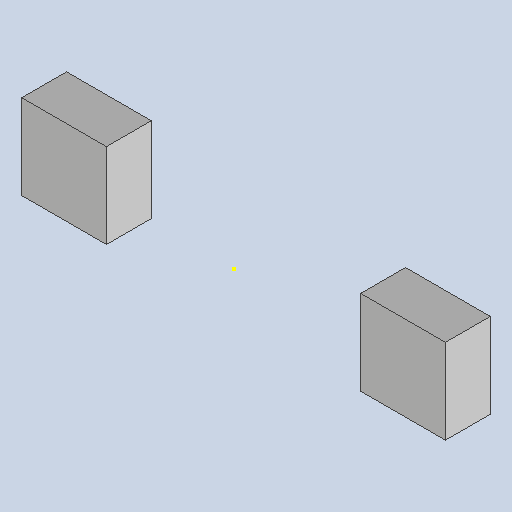
# Autodesk Inventor part: Dots2
Saved by Autodesk Inventor 2024.2 (Build 282272000, 272)
## iProperties
Created: 2024-01-22
Part Number: Dots2
Material: Generic
Document SubType Name: Modeling
Designer: Felix
Density: 1 g/cm^3
Appearance: Default
Author: Felix
Autodesk Inventor part; units mm, degrees
ref_plane "YZ Plane" through (0, 0, 0) normal (1, 0, 0) x (0, 1, 0)
ref_plane "XZ Plane" through (0, 0, 0) normal (0, 1, 0) x (-1, 0, 0)
ref_plane "XY Plane" through (0, 0, 0) normal (0, 0, 1) x (1, 0, 0)
sketch "Sketch1" plane through (0, 0, 0) normal (0, 1, 0) x (-1, 0, 0)
  point P0 (0, 0)
sketch "Sketch2" plane through (0, 0, 0) normal (0, 1, 0) x (-1, 0, 0)
  line L0 (42.5, 8.5) -> (25.5, 8.5)
  line L1 (25.5, 8.5) -> (25.5, -8.5)
  line L2 (25.5, -8.5) -> (42.5, -8.5)
  line L3 (42.5, -8.5) -> (42.5, 8.5)
  line L4 (42.5, 8.5) -> (25.5, -8.5) construction
  line L5 (25.5, 8.5) -> (42.5, -8.5) construction
  line L6 (-25.5, 8.5) -> (-42.5, 8.5)
  line L7 (-42.5, 8.5) -> (-42.5, -8.5)
  line L8 (-42.5, -8.5) -> (-25.5, -8.5)
  line L9 (-25.5, -8.5) -> (-25.5, 8.5)
  line L10 (-25.5, 8.5) -> (-42.5, -8.5) construction
  line L11 (-42.5, 8.5) -> (-25.5, -8.5) construction
  line L12 (0, 0) -> (0, -25.604) construction
  point P0 (34, 0)
  point P1 (-34, 0)
  dimension "d0" = 17
  dimension "d1" = 17
  dimension "d2" = 17
  dimension "d3" = 17
  dimension "d4" = 51
  constraints: 26 end point, 4 midpoint, 4 parallel, 2 horizontal, 2 horizontal alignment, 2 perpendicular, 1 symmetric about line, 1 vertical
  measures "d0" distance of L7.end L8.end
  measures "d1" distance of L6.end L7.end
  measures "d2" distance of L0.end L1.end
  measures "d3" distance of L1.end L2.end
  measures "d4" distance between parallel lines of L9 L1
extrude "Extrusion1" add sketch "Sketch2" along normal blind 9
equation "\"d2\" = d1"
equation "\"d3\" = d0"
body "Solid1"
